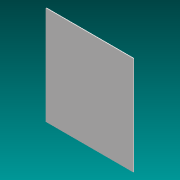
# Autodesk Inventor part: 玻纤板2
Saved by Autodesk Inventor 2021 (Build 250183000, 183)
## iProperties
Created: 2025-04-16
Part Number: 玻纤板2
Material: 常规
Document SubType Name: Modeling
Designer: 86155
Density: 1 g/cm^3
Appearance: 默认
Author: 86155
Autodesk Inventor part; units mm, degrees
ref_plane "YZ Plane" through (0, 0, 0) normal (1, 0, 0) x (0, 1, 0)
ref_plane "XZ Plane" through (0, 0, 0) normal (0, 1, 0) x (-1, 0, 0)
ref_plane "XY Plane" through (0, 0, 0) normal (0, 0, 1) x (1, 0, 0)
sketch "草图1" plane through (0, 0, 0) normal (0, 0, 1) x (1, 0, 0)
  line L0 (0, 0) -> (792, 0)
  line L1 (792, 0) -> (792, -892)
  line L2 (792, -892) -> (0, -892)
  line L3 (0, -892) -> (0, 0)
  dimension "d0" = 792
  dimension "d1" = 892
  constraints: 8 end point, 2 parallel, 1 horizontal, 1 perpendicular
  measures "d0" distance of L1.end L2.end
  measures "d1" distance of L0.end L1.end
extrude "拉伸1" add sketch "草图1" along normal blind 7.6
